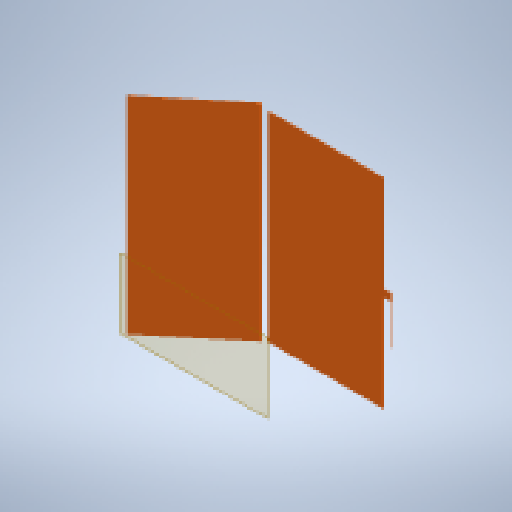
# Autodesk Inventor part: wrapping paper
Saved by Autodesk Inventor 2025 (Build 290162000, 162)
## iProperties
Created: 2024-09-08
Part Number: wrapping paper
Material: Generic
Document SubType Name: Modeling
Designer: Win
Density: 1 g/cm^3
Appearance: Smooth - Light Orange
Author: Win
Autodesk Inventor part; units mm, degrees
ref_plane "YZ Plane" through (0, 0, 0) normal (1, 0, 0) x (0, 1, 0)
ref_plane "XZ Plane" through (0, 0, 0) normal (0, 1, 0) x (-1, 0, 0)
ref_plane "XY Plane" through (0, 0, 0) normal (0, 0, 1) x (1, 0, 0)
ref_plane "Work Plane1" through (0, 81.2927, 0) normal (0, 0, 1) x (1, 0, 0)
sketch "Sketch1" plane through (0, 81.2927, 0) normal (0, 0, 1) x (1, 0, 0)
  line L0 (-965.2, -459.6259) -> (965.2, 403.9741) projected
  line L1 (-965.2, -1501.2668) -> (-965.2, 835.5332) projected
  line L2 (-965.2, 835.5332) -> (-1016, 835.5332) projected
  line L3 (-1016, 835.5332) -> (-1016, -1501.2668) projected
  line L4 (-1016, -1501.2668) -> (-965.2, -1501.2668) projected
  line L5 (-965.2, 2511.9332) -> (-1016, 2459.0165) projected
  line L6 (-1016, 2459.0165) -> (-1016, 835.5332) projected
  line L7 (-1016, 835.5332) -> (-965.2, 835.5332) projected
  line L8 (-965.2, 835.5332) -> (-965.2, 2511.9332) projected
  line L9 (965.2, 3319.8814) -> (965.2, 3375.5332) projected
  line L10 (965.2, 3375.5332) -> (-965.2, 2511.9332) projected
  line L11 (-965.2, 2511.9332) -> (-965.2, 2456.2814) projected
  line L12 (-965.2, 2456.2814) -> (965.2, 3319.8814) projected
  line L13 (965.2, 327.5332) -> (1016, 327.5332) projected
  line L14 (1016, 327.5332) -> (1016, 3375.5332) projected
  line L15 (965.2, 3375.5332) -> (1016, 3375.5332) projected
  line L16 (965.2, 327.5332) -> (965.2, 3375.5332) projected
  line L17 (1016, 327.5332) -> (1066.8, 327.5332) projected
  line L18 (1066.8, 327.5332) -> (1066.8, 3375.5332) projected
  line L19 (1016, 3375.5332) -> (1066.8, 3375.5332) projected
  line L20 (1016, 327.5332) -> (1016, 3375.5332) projected
  line L21 (1066.8, 3375.5332) -> (1066.8, 3273.9332) projected
  line L22 (1066.8, 3273.9332) -> (2743.2, 3273.9332) projected
  line L23 (2743.2, 3375.5332) -> (2743.2, 3273.9332) projected
  line L24 (1066.8, 3375.5332) -> (2743.2, 3375.5332) projected
  line L25 (2844.8, 3273.9332) -> (2743.2, 3273.9332) projected
  line L26 (2743.2, 3273.9332) -> (2743.2, 1876.9332) projected
  line L27 (2844.8, 1876.9332) -> (2743.2, 1876.9332) projected
  line L28 (2844.8, 3273.9332) -> (2844.8, 1876.9332) projected
  line L29 (2836.6524, 1775.3332) -> (2735.0524, 1775.3332) projected
  line L30 (2735.0524, 1775.3332) -> (2735.0524, 378.3332) projected
  line L31 (2836.6524, 378.3332) -> (2735.0524, 378.3332) projected
  line L32 (2836.6524, 1775.3332) -> (2836.6524, 378.3332) projected
  line L33 (2844.8, 276.7332) -> (2743.2, 276.7332) projected
  line L34 (2743.2, 276.7332) -> (2743.2, -1399.6668) projected
  line L35 (2844.8, -1399.6668) -> (2743.2, -1399.6668) projected
  line L36 (2844.8, 276.7332) -> (2844.8, -1399.6668) projected
  line L37 (2743.2, -1399.6668) -> (2844.8, -1399.6668) projected
  line L38 (2743.2, -1501.2668) -> (2743.2, -1399.6668) projected
  line L39 (2844.8, -1501.2668) -> (2743.2, -1501.2668) projected
  line L40 (2844.8, -1399.6668) -> (2844.8, -1501.2668) projected
  line L41 (1066.8, -1399.6668) -> (1066.8, -1501.2668) projected
  line L42 (1066.8, -1501.2668) -> (2743.2, -1501.2668) projected
  line L43 (2743.2, -1399.6668) -> (2743.2, -1501.2668) projected
  line L44 (1066.8, -1399.6668) -> (2743.2, -1399.6668) projected
  line L45 (965.2, -1399.6668) -> (-965.2, -1399.6668) projected
  line L46 (-965.2, -1399.6668) -> (-965.2, -1501.2668) projected
  line L47 (-965.2, -1501.2668) -> (965.2, -1501.2668) projected
  line L48 (965.2, -1501.2668) -> (965.2, -1399.6668) projected
  line L49 (-1016, -1501.2668) -> (-1016, 2459.0165)
  line L50 (-965.2, 2511.9332) -> (-1016, 2459.0165)
  line L51 (-965.2, 2511.9332) -> (965.2, 3375.5332)
  line L52 (2743.2, 276.7332) -> (2844.8, 276.7332) projected
  line L53 (2844.8, 276.7332) -> (2844.8, 1191.1332) projected
  line L54 (2743.2, 1191.1332) -> (2844.8, 1191.1332) projected
  line L55 (2743.2, 276.7332) -> (2743.2, 1191.1332) projected
  line L56 (2133.6, 378.3332) -> (2133.6, 276.7332) projected
  line L57 (2133.6, 276.7332) -> (2743.2, 276.7332) projected
  line L58 (2743.2, 378.3332) -> (2743.2, 276.7332) projected
  line L59 (2133.6, 378.3332) -> (2743.2, 378.3332) projected
  line L60 (1066.8, 378.3332) -> (1066.8, 276.7332) projected
  line L61 (1066.8, 276.7332) -> (2743.2, 276.7332) projected
  line L62 (2743.2, 378.3332) -> (2743.2, 276.7332) projected
  line L63 (1066.8, 378.3332) -> (2743.2, 378.3332) projected
  line L64 (-965.2, -459.6259) -> (-1016, -459.6259)
  line L65 (-965.2, -459.6259) -> (965.2, 327.5332)
  line L66 (965.2, 327.5332) -> (2844.8, 327.5332)
  line L67 (2844.8, 327.5332) -> (2844.8, 3375.5332)
  line L68 (2844.8, 3375.5332) -> (965.2, 3375.5332)
  line L69 (965.2, 3375.5332) -> (-965.2, 2511.9332)
  line L70 (-965.2, 2511.9332) -> (-1016, 2459.0165)
  line L71 (-1016, 2459.0165) -> (-1016, -459.6259)
  line L72 (965.2, 327.5332) -> (1016, 327.5332) projected
  line L73 (1016, 327.5332) -> (1016, 3375.5332) projected
  line L74 (965.2, 3375.5332) -> (1016, 3375.5332) projected
  line L75 (965.2, 327.5332) -> (965.2, 3375.5332) projected
  line L76 (1016, 327.5332) -> (1066.8, 327.5332) projected
  line L77 (1066.8, 327.5332) -> (1066.8, 3375.5332) projected
  line L78 (1016, 3375.5332) -> (1066.8, 3375.5332) projected
  line L79 (1016, 327.5332) -> (1016, 3375.5332) projected
  point P0 (0, -81.2927)
  point P1 (1066.8, 459.6259)
  point P2 (2735.0524, 378.3332)
  point P3 (2836.6524, 1191.1332)
  point P4 (2844.8, 1191.1332)
  point P5 (2844.8, 1876.9332)
  point P6 (-965.2, -459.6259)
  point P7 (965.2, 3401.1741)
  point P8 (2743.2, 378.3332)
  point P9 (2743.2, 327.5332)
  point P10 (2133.6, 327.5332)
  constraints: 22 end point, 5 collinear, 4 point on line, 2 parallel, 1 perpendicular
extrude "Extrusion1" add sketch "Sketch1" along normal blind 6.35 contours L1 L8 L12 L16 L0 | L64 L3 L2 L1 | L1 L4 L3 L64 | L0 L16 L65 | L16 L9 L15 L14 L13 | L2 L6 L5 L8 | L12 L8 L10 L9 | L14 L19 L18 L17 | L24 L23 L22 L18 | L18 L22 L26 L27 L67 L54 L32 L29 L30 L59 L63 | L56 L59 L31 L55 L66 | L68 L67 L25 L23 | L66 L53 L33 L55 | L55 L31 L32 L54 L53 L66 | L25 L28 L27 L26 | L30 L29 L32 L54 L55 L31 | L55 L54 L32 L31
body "Solid1"
